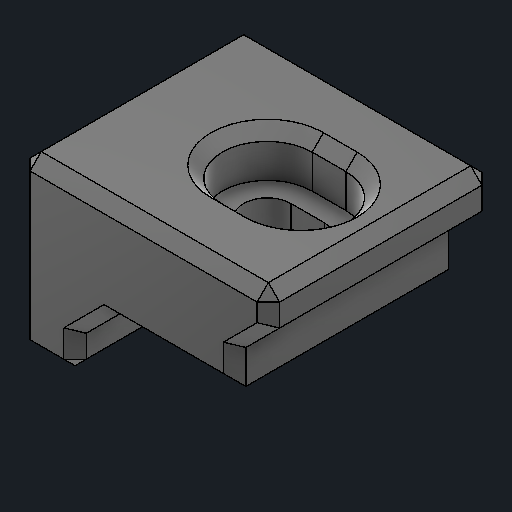
# Autodesk Inventor part: Moving Jaw (M4) Normal
Saved by Autodesk Inventor 2026.2 (Build 302298000, 298)
## iProperties
Created: 2026-07-19
Part Number: Moving Jaw (M4) Normal
Material: ABS Plastic
Document SubType Name: Modeling
Designer: JoshuaEah
Density: 1.06 g/cm^3
Appearance: Smooth - Black
Author: JoshuaEah
Autodesk Inventor part; units mm, degrees
ref_plane "YZ Plane" through (0, 0, 0) normal (1, 0, 0) x (0, 1, 0)
ref_plane "XZ Plane" through (0, 0, 0) normal (0, 1, 0) x (-1, 0, 0)
ref_plane "XY Plane" through (0, 0, 0) normal (0, 0, 1) x (1, 0, 0)
sketch "Base Sketch" plane through (0, 0, 0) normal (0, 0, 1) x (1, 0, 0)
  line L0 (0, 0) -> (5, 0)
  line L1 (5, 0) -> (5, 3)
  line L2 (5, 3) -> (8, 6)
  line L3 (8, 6) -> (19.2, 6)
  line L4 (22.2, 15) -> (0, 15)
  line L5 (0, 15) -> (0, 0)
  line L6 (19.2, 6) -> (19.2, 9)
  line L7 (19.2, 9) -> (22.2, 12)
  line L8 (22.2, 12) -> (22.2, 15)
  dimension "d0" = 45
  dimension "d2" = 5
  dimension "d4" = 11.2
  dimension "d7" = 3
  dimension "d32" = 3
  dimension "d45" = 3
  dimension "d47" = 3
  constraints: 18 end point, 3 parallel, 2 perpendicular, 2 vertical, 1 coincident, 1 horizontal
  measures "d0" angle of L2 L1
  measures "d2" distance between parallel lines of L1 L5
  measures "d4" distance of L2.end L3.end
  measures "d7" distance of L0.end L1.end
  measures "d32" horizontal distance of L1.end L2.end
  measures "d45" distance of L7.end L4.start
  measures "d47" distance of L3.end L6.end
extrude "Profile" add sketch "Base Sketch" along normal blind 20
sketch "CB Slot Sketch" plane through (0, 15, 0) normal (0, 1, 0) x (1, 0, 0)
  line L0 (10, -10) -> (17.2, -10) construction
  line L1 (12.1, -12.1) -> (15.1, -12.1)
  line L2 (15.1, -7.9) -> (12.1, -7.9)
  arc A0 (12.1, -7.9) -> (12.1, -12.1) centre (12.1, -10) ccw
  arc A1 (15.1, -12.1) -> (15.1, -7.9) centre (15.1, -10) ccw
  line L3 (12.1, -10) -> (15.1, -10) construction
  line L4 (12.1, -14.0005) -> (15.1, -14.0005)
  line L5 (15.1, -5.9995) -> (12.1, -5.9995)
  arc A2 (12.1, -5.9995) -> (12.1, -14.0005) centre (12.1, -10) ccw
  arc A3 (15.1, -14.0005) -> (15.1, -5.9995) centre (15.1, -10) ccw
  line L6 (8, 0) -> (19.2, 0) construction
  line L7 (19.2, 0) -> (19.2, -20) construction
  line L8 (8, -20) -> (19.2, -20) construction
  line L9 (8, 0) -> (8, -20) construction
  point P0 (13.6, -10)
  point P1 (10, -10)
  point P2 (8.0995, -10)
  point P3 (13.6, -20)
  point P4 (8, -10)
  dimension "d11" = 4.2
  dimension "d16" = 8.001
  dimension "d24" = 3
  constraints: 16 end point, 13 point on circle, 8 tangent, 4 centre point, 4 midpoint, 3 point on line, 2 parallel, 1 coincident, 1 horizontal, 1 horizontal alignment, 1 vertical alignment
  measures "d11" diameter of A1
  measures "d16" diameter of A3
  measures "d24" distance of L3.end A0.centre
extrude "M4 Slot" cut sketch "CB Slot Sketch" against normal through all contours A0 L2 A1 L1
extrude "M4 CB Slot" cut sketch "CB Slot Sketch" against normal blind 4 contours A0 L2 A1 L1 | A2 L5 A3 L4
sketch "Inset Pattern" plane through (0, 0, 0) normal (-1, 0, 0) x (0, 0, 1)
  line L0 (0, 15) -> (0, 0) construction
  line L1 (0, 0) -> (20, 0) construction
  line L2 (20, 15) -> (20, 0) construction
  line L3 (0, 15) -> (20, 15) construction
  line L4 (2.5, 12.5) -> (17.5, 12.5)
  line L5 (17.5, 12.5) -> (17.5, 2.5)
  line L6 (17.5, 2.5) -> (2.5, 2.5)
  line L7 (2.5, 2.5) -> (2.5, 12.5)
  point P0 (17.5, 7.5)
  point P1 (20, 7.5)
  point P2 (10, 12.5)
  point P3 (10, 15)
  dimension "d48" = 15
  dimension "d49" = 10
  constraints: 8 end point, 4 midpoint, 2 parallel, 1 horizontal, 1 horizontal alignment, 1 perpendicular, 1 vertical alignment
  measures "d48" distance of L4.start L4.end
  measures "d49" distance of L6.end L4.start
extrude "Inset" cut sketch "Inset Pattern" against normal blind 0.5
chamfer "Inset Chamfer" distance 0.5 angle 45 4 edges at (0, 12.5, 10) (0, 7.5, 17.5) (0, 7.5, 2.5) (0, 2.5, 10)
chamfer "Edgebreak" distance 1 angle 45 26 edges at (11.1, 15, 20) (11.1, 15, 0) (0, 15, 10) (0, 7.5, 20) (0, 7.5, 0) (0, 0, 10) (2.5, 0, 20) (2.5, 0, 0) (20.7, 10.5, 20) (19.2, 7.5, 20) (13.6, 6, 20) (6.5, 4.5, 20) (5, 1.5, 20) (5, 1.5, 0) (6.5, 4.5, 0) (13.6, 6, 0) (19.2, 7.5, 0) (20.7, 10.5, 0) (19.1005, 15, 10) (13.6, 15, 14.0005) (8.0995, 15, 10) (13.6, 15, 5.9995) (22.2, 13.5, 20) (22.2, 13.5, 0) (22.2, 15, 10) (5, 0, 10)
equation "\"d7\" = d6"
equation "\"d24\" = jawTravel"
equation "\"jawTravel\" = 3"
equation "\"slotLength\" = M4_clearance_hole + jawTravel"
equation "\"M4_clearance_hole\" = 4.2"
equation "\"chamferSize\" = 1"
equation "\"jawThickness\" = 5"
equation "\"topThickness\" = 3"
equation "\"d6\" = 3"
body "Solid1"
